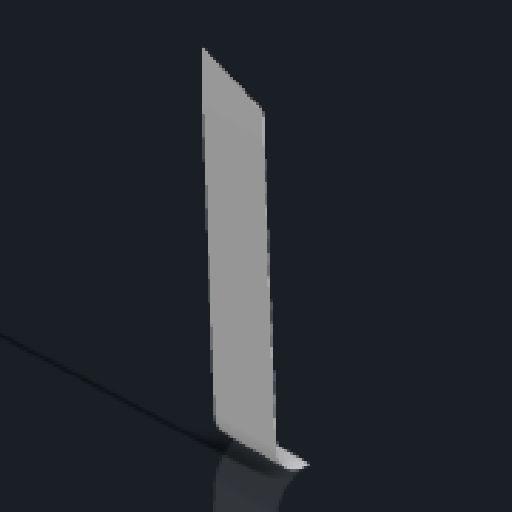
# Autodesk Inventor part: CARCASA_ALUM_3
Saved by Autodesk Inventor 2024.3 (Build 283343000, 343)
## iProperties
Created: 2024-05-14
Part Number: CARCASA_ALUM_3
Material: Generic
Document SubType Name: Sheet Metal
Designer: Niler
Density: 1 g/cm^3
Sheet Metal Rule: Default_mm
Appearance: Default
Flat Pattern Width: 22 cm
Flat Pattern Length: 133.058 cm
Flat Pattern Area: 2927.28 cm^2
Sheet Metal Width: 220.000 mm
Sheet Metal Length: 1330.583 mm
Sheet Metal Area: 292728.302 mm^2
Author: Niler
Autodesk Inventor part; units mm, degrees
ref_plane "Work Plane6" through (0, -199.5457, 0) normal (0, -0.0454077, 0.9989685) x (1, 0, 0)
sketch "Sketch4" plane through (0, -199.5457, 0) normal (0, -0.0454077, 0.9989685) x (1, 0, 0)
  line L0 (220, 0) -> (220, -976.9106)
  line L1 (0, 0) -> (220, 0)
  line L2 (0, 0) -> (0, -976.9106)
  line L3 (0, -976.9106) -> (220, -976.9106)
  point P0 (0, 199.3399)
extrude "Plate4" add sketch "Sketch4" against normal blind 1.5
ref_plane "Work Plane7" through (0, 0, 0) normal (0, 0, 1) x (1, 0, 0)
sketch "Sketch5" plane through (0, 0, 0) normal (0, 0, -1) x (1, 0, 0)
  line L0 (0, -166.5116) -> (220, -166.5116)
  line L1 (220, -166.5116) -> (220, 0.4543)
  line L2 (220, 0.4543) -> (0, 0.4543)
  line L3 (0, 0.4543) -> (0, -166.5116)
  constraints: 8 end point
edge flange "Flange3" height 200 angle 90 thickness 1.5 bend radius 1.5 thickness toward (0, 0, -1) relief tear relief width 1.5 relief depth 0.75 edges at (110, -199.4776, -1.4985) wall of the first edge with corners at (0, -166.5116, 0) (220, -166.5116, 0) (220, 0.4543, 0) (0, 0.4543, 0)
bend "Bend3"
corner "Corner3"
sketch "Sketch6" plane through (0, 0.4543, 0) normal (0, 0, 1) x (1, 0, 0)
  arc A0 (220, -130.306) -> (201.1417, -102.4517) centre (190, -130.306) ccw projected
  line L0 (0, -21.995) -> (201.1417, -102.4517) projected
  line L1 (0, -21.995) -> (0, -200) projected
  line L2 (0, -200) -> (220, -200) projected
  line L3 (220, -130.306) -> (220, -200) projected
  line L4 (0, -199.9319) -> (220, -199.9319) projected
  line L5 (220, 0) -> (220, -199.9319) projected
  line L6 (0, 0) -> (220, 0) projected
  line L7 (0, -199.9319) -> (0, 0) projected
  point P0 (0, -0.4543)
  point P1 (220, -130.306)
extrude "Extrusion1" cut sketch "Sketch6" against normal through all contours A0 L0 L7 L6 L5
ref_plane "Work Plane9" through (125, -1279.7641, -134.7549) normal (0, -1, 0) x (-1, 0, 0)
sketch "Sketch8" plane through (125, -1279.7641, -134.7549) normal (0, 1, 0) x (-1, 0, 0)
  line L0 (-95, -84.1525) -> (125, -84.1525)
  line L1 (125, -84.1525) -> (125, 29.3459)
  line L2 (125, 29.3459) -> (-95, 29.3459)
  line L3 (-95, 29.3459) -> (-95, -84.1525)
  constraints: 8 end point
edge flange "Flange5" height 115 angle 90 thickness 1.5 bend radius 108.5 thickness toward (0, 1, 0) relief tear relief width 1.5 relief depth 0.75 edges at (110, -1175.3806, -45.8577) wall of the first edge with corners at (220, -1279.7641, -50.6024) (0, -1279.7641, -50.6024) (0, -1279.7641, -164.1008) (220, -1279.7641, -164.1008)
bend "Bend5"
corner "Corner5"
ref_plane "Work Plane8" through (125, -1278.2641, -134.7549) normal (0, -1, 0) x (-1, 0, 0)
sketch "Sketch9" plane through (220, -1279.7641, -164.1008) normal (1, 0, 0) x (0, 0, -1)
  line L0 (-9.8864, 1.5) -> (-9.8864, 0) projected
  arc A0 (-118.2745, 105.0733) -> (-9.8864, 1.5) centre (-9.8864, 110) ccw projected
  line L1 (-119.773, 105.0052) -> (-118.2745, 105.0733) projected
  arc A1 (-119.773, 105.0052) -> (-9.8864, 0) centre (-9.8864, 110) ccw projected
  line L2 (-9.8864, 1.5) -> (-9.8864, 0) projected
  line L3 (-9.8864, 0) -> (0, 0) projected
  line L4 (0, 1.5) -> (0, 0) projected
  line L5 (-9.8864, 1.5) -> (0, 1.5) projected
  line L6 (-29.3211, 1.7305) -> (-29.0561, 3.2069)
  point P0 (-164.1008, 1279.7641)
  constraints: 2 end point, 2 line through centre, 2 point on circle
sketch3d "3D Sketch1"
sketch "Sketch1" plane through (0, 0, 0) normal (0, 0, 1) x (1, 0, 0)
  line L0 (1250.1265, -201.1417) -> (1330.5832, 0) projected
  line L1 (0, 0) -> (1330.5832, 0) projected
  line L2 (0, -220) -> (0, 0) projected
  line L3 (1222.2722, -220) -> (0, -220) projected
  arc A0 (1222.2722, -220) -> (1250.1265, -201.1417) centre (1222.2722, -190) ccw projected
equation "\"d22\" = Thickness"
equation "\"d23\" = BendReliefWidth"
equation "\"d24\" = BendReliefDepth"
equation "\"d25\" = MinimumRemnant"
equation "\"d26\" = TransitionRadius"
equation "\"d29\" = BendRadius"
equation "\"d30\" = CornerReliefSize"
equation "\"d31\" = GapSize"
equation "\"d32\" = JacobiRadiusSize"
equation "\"d46\" = BendReliefWidth"
equation "\"d47\" = BendReliefDepth"
equation "\"d48\" = MinimumRemnant"
equation "\"d49\" = TransitionRadius"
equation "\"d53\" = CornerReliefSize"
equation "\"d54\" = GapSize"
equation "\"d55\" = JacobiRadiusSize"
equation "\"BendRadius\" = Thickness"
equation "\"BendReliefWidth\" = Thickness"
equation "\"BendReliefDepth\" = 0.5 * Thickness"
equation "\"CornerReliefSize\" = 4 * Thickness"
equation "\"MinimumRemnant\" = 2 * Thickness"
equation "\"TransitionRadius\" = BendRadius"
equation "\"JacobiRadiusSize\" = BendRadius"
equation "\"GapSize\" = Thickness"
equation "\"Thickness\" = 1.5"
body "Solid2"
